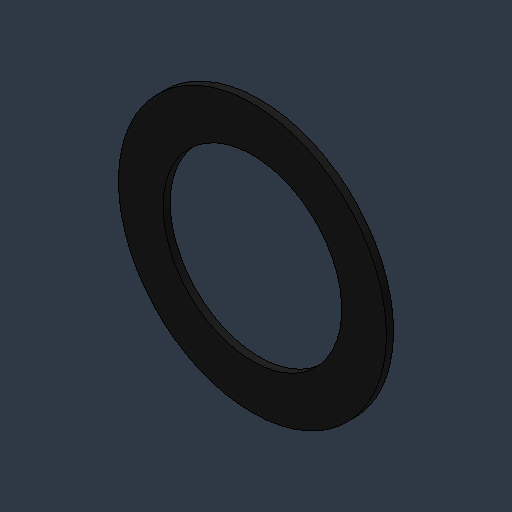
# Autodesk Inventor part: SPACER,BEARING,SLIDE,THIN,ELEVATOR
Saved by Autodesk Inventor 2024.3 (Build 283343000, 343)
## iProperties
Category: _
Manager: _
ILogicPurgeVersion: 0.0.0.0
OnSaveVersion: 3.4.3.0
OnSaveAssembly: COREAutomationManager
Created: 2025-01-27
Part Number: SPACER,BEARING,SLIDE,THIN,ELEVATOR
Checked By: 00
Engr Approved By: _
User Status: Work In Process
Material: 3D Print Material - chopped carbon Nylon12 (preferred)
Description: STANDARD (mm)
Document SubType Name: Modeling
Mfg Approved By: John.Thibert
Designer: John.Thibert
Manufacturer: Standard
Standards Organization: Custom
Density: 1.05184 g/cm^3
Appearance: Black
Mass: 0.0105762 g
Surface Area: 0.918407 cm^2
Volume: 0.010055 cm^3
CN_MASS: 0.0
CN_SERVICEABLE: _
FIRST_DESCRIPTION: _
SECOND_DESCRIPTION: _
THIRD_DESCRIPTION: _
ModelCat: Uncategorized
MaterialName: 3D Print Material - chopped carbon Nylon12 (preferred)
Subject: _
Author: John.Thibert
Keywords: -
Revision Number: A
Autodesk Inventor part; units mm, degrees
ref_plane "YZ Plane" through (0, 0, 0) normal (1, 0, 0) x (0, 1, 0)
ref_plane "XZ Plane" through (0, 0, 0) normal (0, 1, 0) x (-1, 0, 0)
ref_plane "XY Plane" through (0, 0, 0) normal (0, 0, 1) x (1, 0, 0)
sketch "Sketch2" plane through (0, 0, 0) normal (0, 1, 0) x (-1, 0, 0)
  line L0 (3.175, -0.127) -> (3.175, 0.127)
  line L1 (3.175, 0.127) -> (4.7625, 0.127)
  line L2 (4.7625, 0.127) -> (4.7625, -0.127)
  line L3 (4.7625, -0.127) -> (3.175, -0.127)
  line L4 (0, -0.1778) -> (0, 0.1778) construction
  point P0 (0, 0)
  point P1 (3.175, 0)
  dimension "d0" = 6.35
  dimension "d1" = 9.525
  dimension "d2" = 0.254
  constraints: 8 end point, 3 perpendicular, 1 horizontal alignment, 1 midpoint, 1 vertical
  measures "d0" diameter of L0 L4
  measures "d1" diameter of L2 L4
  measures "d2" distance of L1.end L2.end
revolve "Revolution1" add sketch "Sketch2" angle 360 about axis through (0, 0, -10) along (0, 0, 1)
body "Solid1"
